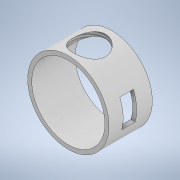
# Autodesk Inventor part: Cadran base
Saved by Autodesk Inventor 2021 (Build 250183000, 183)
## iProperties
Created: 2020-09-18
Part Number: Cadran base
Material: Générique
Document SubType Name: Modeling
Designer: Utilisateur
Density: 1 g/cm^3
Appearance: Par défaut
Author: Utilisateur
Autodesk Inventor part; units mm, degrees
ref_plane "YZ Plane" through (0, 0, 0) normal (1, 0, 0) x (0, 1, 0)
ref_plane "XZ Plane" through (0, 0, 0) normal (0, 1, 0) x (-1, 0, 0)
ref_plane "XY Plane" through (0, 0, 0) normal (0, 0, 1) x (1, 0, 0)
sketch "Esquisse1" plane through (0, 0, 0) normal (0, 0, 1) x (1, 0, 0)
  circle A0 centre (0, 0) radius 30
  circle A1 centre (0, 0) radius 27
  dimension "d0" = 60
  dimension "d1" = 54
  constraints: 2 centre point, 2 coincident
  measures "d0" diameter of A0
  measures "d1" diameter of A1
extrude "Extrusion1" add sketch "Esquisse1" along normal blind 32
sketch "Esquisse2" plane through (0, 0, 0) normal (0, 1, 0) x (-1, 0, 0)
  circle A0 centre (0, 16.4966) radius 15.5
  circle A1 centre (0, 16.4966) radius 12
  point P0 (0, 0)
  dimension "d18" = 24
  dimension "d19" = 31
  constraints: 2 centre point, 1 coincident
  measures "d18" diameter of A1
  measures "d19" diameter of A0
extrude "Extrusion2" cut sketch "Esquisse2" along normal blind 111.75 contours A1
thread "Filetage1" size "M25x2" class "6H" standard "ANSI Metric M Profile" full length
sketch "Esquisse3" plane through (0, 0, 0) normal (1, 0, 0) x (0, 1, 0)
  line L0 (11.9576, 21.526) -> (-8.0424, 21.526)
  line L1 (-8.0424, 21.526) -> (-8.0424, 11.526)
  line L2 (-8.0424, 11.526) -> (11.9576, 11.526)
  line L3 (11.9576, 11.526) -> (11.9576, 21.526)
  line L4 (0, 0) -> (0, 32)
  line L5 (30, 0) -> (-30, 0) projected
  dimension "d10" = 10
  dimension "d12" = 32
  dimension "d17" = 20
  constraints: 10 end point, 2 parallel, 2 perpendicular, 1 horizontal
  measures "d10" distance of L2.end L0.start
  measures "d12" distance of L4.start L4.end
  measures "d17" distance of L0.start L0.end
extrude "Extrusion3" cut sketch "Esquisse3" along normal blind 30
